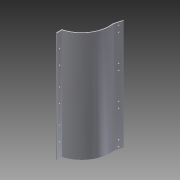
# Autodesk Inventor part: 装填斗后罩
Saved by Autodesk Inventor 2015 (Build 190159000, 159)
## iProperties
Created: 2017-05-04
Part Number: 装填斗后罩
Material: 常规
Document SubType Name: Modeling
Designer: Administrator
Density: 1 g/cm^3
Appearance: 雪
Author: Administrator
Autodesk Inventor part; units mm, degrees
ref_plane "YZ Plane" through (0, 0, 0) normal (1, 0, 0) x (0, 1, 0)
ref_plane "XZ Plane" through (0, 0, 0) normal (0, 1, 0) x (-1, 0, 0)
ref_plane "XY Plane" through (0, 0, 0) normal (0, 0, 1) x (1, 0, 0)
sketch "草图1" plane through (0, 0, 0) normal (0, 0, 1) x (1, 0, 0)
  circle A0 centre (0, 0) radius 100
  line L0 (-25, -96.8246) -> (25, -96.8246)
  line L1 (25, -96.8246) -> (25, -118)
  line L2 (25, -118) -> (-25, -118)
  line L3 (-25, -118) -> (-25, -96.8246)
  line L4 (0, -100) -> (-25, -100)
  arc A1 (28, -99.1211) -> (102.0345, 14.0701) centre (0, 0) ccw
  line L5 (25, -118) -> (28, -118)
  line L6 (28, -118) -> (28, -99.1211)
  line L7 (98.9752, 14.2797) -> (107.1784, 43.1364)
  line L8 (107.1784, 43.1364) -> (110.0641, 42.3161)
  line L9 (110.0641, 42.3161) -> (102.0345, 14.0701)
  line L10 (-25, 96.8246) -> (-25, 300)
  line L11 (-25, 300) -> (175, 300)
  line L12 (175, 300) -> (96.8246, 25)
  dimension "d0" = 200
  dimension "d1" = 50
  dimension "d2" = 18
  dimension "d3" = 3
  dimension "d4" = 3
  dimension "d5" = 3
  dimension "d6" = 200
  dimension "d7" = 25
  dimension "d8" = 25
  dimension "d9" = 5
  dimension "d10" = 300
  dimension "d11" = 30
  constraints: 26 end point, 8 point on circle, 6 perpendicular, 3 parallel, 2 centre point, 2 horizontal, 1 coincident, 1 concentric, 1 point on line, 1 tangent, 1 vertical
  measures "d0" diameter of A0
  measures "d1" distance of L0.start L0.end
  measures "d2" distance between parallel lines of L2 L4
  measures "d3" radial gap between concentric circles of A0 A1
  measures "d4" distance of L1.end L5.end
  measures "d5" distance between parallel lines of L9 L7
  measures "d6" distance of L10.end L11.end
  measures "d7" horizontal distance of point (0, 0) L10.start
  measures "d8" vertical distance of point (0, 0) L12.end
  measures "d9" distance between parallel lines of L7 L12
  measures "d10" distance from line of point (0, 0) L11
  measures "d11" distance from line of L8 L7.start
extrude "拉伸1" add sketch "草图1" against normal blind 398 contours A0 L7 L8 L9 A1 L6 L5 L1
sketch "草图2" plane through (28, -118, 0) normal (1, 0, 0) x (0, 0, -1)
  circle A0 centre (293, 10) radius 2.5
  circle A1 centre (345, 10) radius 2.5
  line L0 (0, 0) -> (398, 0) projected
  line L1 (398, 18.8789) -> (398, 0) projected
  point P0 (0, 118)
  dimension "d14" = 5
  dimension "d15" = 5
  dimension "d16" = 10
  dimension "d17" = 10
  dimension "d18" = 53
  dimension "d19" = 105
  constraints: 2 centre point
  measures "d14" diameter of A0
  measures "d15" diameter of A1
  measures "d16" distance from line of L0 A1.centre
  measures "d17" distance from line of L0 A0.centre
  measures "d18" distance from line of L1 A1.centre
  measures "d19" distance from line of L1 A0.centre
extrude "拉伸2" cut sketch "草图2" against normal blind 3
pattern_linear "矩形阵列1" count 3 spacing 120 along (0, 0, 1) of "拉伸2"
sketch "草图3" plane through (102.0345, 14.0701, 0) normal (0.9619, -0.2734, 0) x (0, 0, -1)
  circle A0 centre (390, 14.3651) radius 2.5
  circle A1 centre (368, 14.3651) radius 2.5
  line L0 (0, 29.3651) -> (398, 29.3651) projected
  line L1 (398, 29.3651) -> (398, 0) projected
  point P0 (0, -41.4342)
  dimension "d25" = 5
  dimension "d26" = 5
  dimension "d27" = 15
  dimension "d28" = 15
  dimension "d29" = 8
  dimension "d30" = 30
  constraints: 2 centre point
  measures "d25" diameter of A0
  measures "d26" diameter of A1
  measures "d27" distance from line of L0 A0.centre
  measures "d28" distance from line of L0 A1.centre
  measures "d29" distance from line of L1 A0.centre
  measures "d30" distance from line of L1 A1.centre
extrude "拉伸3" cut sketch "草图3" against normal blind 3
pattern_linear "矩形阵列2" count 4 spacing 120 along (0, 0, 1) of "拉伸3"
